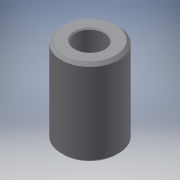
# Autodesk Inventor part: TestPart
Saved by Autodesk Inventor 2016 SP1 (Build 200210100, 210)
## iProperties
Created: 2007-04-12
Part Number: TestPart
Document SubType Name: Modeling
Designer: leefsmp
Density: 1 g/cm^3
Material: Generic
Appearance: Default
Author: leefsmp
Autodesk Inventor part; units mm, degrees
ref_plane "YZ Plane" through (0, 0, 0) normal (1, 0, 0) x (0, 1, 0)
ref_plane "XZ Plane" through (0, 0, 0) normal (0, 1, 0) x (-1, 0, 0)
ref_plane "XY Plane" through (0, 0, 0) normal (0, 0, 1) x (1, 0, 0)
sketch "Sketch1" plane through (0, 0, 0) normal (0, 0, 1) x (1, 0, 0)
  line L0 (-50, 88.8965) -> (-25, 88.8965)
  line L1 (-25, 88.8965) -> (-25, -61.1035)
  line L2 (-25, -61.1035) -> (-50, -61.1035)
  line L3 (-50, -61.1035) -> (-50, 88.8965)
  line L4 (0, 88.8965) -> (0, -88.8965)
  point P0 (0, 0)
  point P1 (0, 0)
  dimension "d10" = 150
  dimension "d12" = 25
  dimension "d13" = 50
  constraints: 10 end point, 3 parallel, 1 coincident, 1 horizontal, 1 horizontal alignment, 1 midpoint, 1 perpendicular
  measures "d10" distance of L2.end L0.start
  measures "d12" distance between parallel lines of L1 L4
  measures "d13" distance between parallel lines of L3 L4
revolve "Revolution1" add sketch "Sketch1" angle 360 about axis through (0, 88.8965, 0) along (0, -1, 0)
chamfer "Chamfer1" distance 2 angle 45 2 edges at (25, 88.8965, 0) (25, -61.1035, 0)
chamfer "Chamfer3" distance 5 angle 45 2 edges at (50, 88.8965, 0) (50, -61.1035, 0)
body "Solid1"
